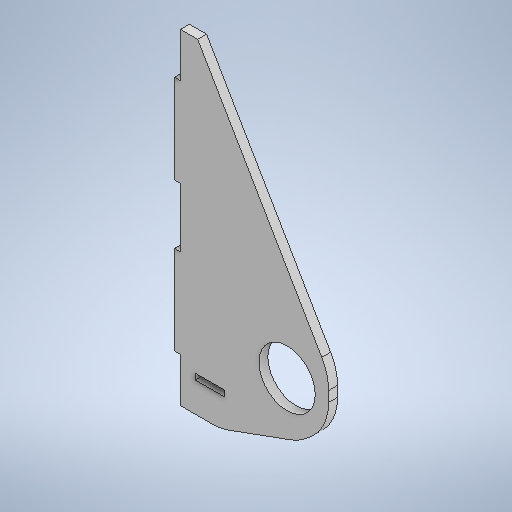
# Autodesk Inventor part: Piston_FloorHinge01
Saved by Autodesk Inventor 2025.2 (Build 292293000, 293)
## iProperties
Created: 2025-04-08
Part Number: Piston_FloorHinge01
Material: Generic
Document SubType Name: Sheet Metal
Designer: Victor
Density: 1 g/cm^3
Sheet Metal Rule: Default_mm
Appearance: Default
Author: Victor
Autodesk Inventor part; units mm, degrees
ref_plane "YZ Plane" through (0, 0, 0) normal (1, 0, 0) x (0, 1, 0)
ref_plane "XZ Plane" through (0, 0, 0) normal (0, 1, 0) x (-1, 0, 0)
ref_plane "XY Plane" through (0, 0, 0) normal (0, 0, 1) x (1, 0, 0)
sketch "Sketch1" plane through (0, 0, 0) normal (0, 0, 1) x (1, 0, 0)
  line L0 (-16.7671, 64.9713) -> (-16.7671, -55.0287)
  line L1 (-16.7671, -55.0287) -> (11.7813, -55.0287)
  line L2 (11.7813, -55.0287) -> (33.2329, -37.0287)
  line L3 (33.2329, -37.0287) -> (33.2329, -21.0287)
  line L4 (33.2329, -21.0287) -> (-16.7671, 64.9713)
  line L5 (-1.7671, -43.0287) -> (-11.7671, -43.0287)
  line L6 (-11.7671, -43.0287) -> (-11.7671, -45.0287)
  line L7 (-11.7671, -45.0287) -> (-1.7671, -45.0287)
  line L8 (-1.7671, -45.0287) -> (-1.7671, -43.0287)
  line L9 (-16.7671, -40.0287) -> (-18.7671, -40.0287)
  line L10 (-18.7671, -40.0287) -> (-18.7671, -10.0287)
  line L11 (-18.7671, -10.0287) -> (-16.7671, -10.0287)
  line L12 (-16.7671, -10.0287) -> (-16.7671, -40.0287)
  line L13 (-16.7671, 9.9713) -> (-18.7671, 9.9713)
  line L14 (-18.7671, 9.9713) -> (-18.7671, 39.9713)
  line L15 (-18.7671, 39.9713) -> (-16.7671, 39.9713)
  line L16 (-16.7671, 39.9713) -> (-16.7671, 9.9713)
  line L17 (-16.7671, 54.9713) -> (-10.9532, 54.9713)
  circle A0 centre (19.2329, -29.0287) radius 9.5
  line L18 (19.2329, -29.0287) -> (33.2329, -29.0287)
  point P0 (0, 0)
  point P1 (-17.7671, -40.0287)
  point P2 (-17.7671, -10.0287)
  dimension "d0" = 120
  dimension "d1" = 10
  dimension "d2" = 2
  dimension "d3" = 10
  dimension "d4" = 5
  dimension "d5" = 2
  dimension "d6" = 30
  dimension "d7" = 15
  dimension "d8" = 2
  dimension "d9" = 30
  dimension "d10" = 20
  dimension "d11" = 18
  dimension "d12" = 16
  dimension "d13" = 50
  dimension "d14" = 10
  dimension "d15" = 50
  dimension "d16" = 19
  dimension "d17" = 36
  dimension "d18" = 90
  measures "d0" distance of L0.start L0.end
  measures "d1" distance of L7.end L7.start
  measures "d2" distance of L7.start L5.end
  measures "d3" distance between parallel lines of L1 L7
  measures "d4" distance between parallel lines of L0 L6
  measures "d5" distance of L11.start L11.end
  measures "d6" distance of L10.start L11.start
  measures "d7" distance from line of L1 point (-17.767, -40.029)
  measures "d8" distance of L14.end L16.start
  measures "d9" distance of L14.start L14.end
  measures "d10" distance from line of point (-17.767, -10.029) L13
  measures "d11" distance from line of L2.end L1
  measures "d12" distance of L2.end L4.start
  measures "d13" distance between parallel lines of L12 L3
  measures "d14" distance from line of L0.start L17
  measures "d15" angle of L0 L2
  measures "d16" diameter of A0
  measures "d17" distance from line of L12 L18.start
  measures "d18" angle of L3 L18
extrude "Plate1" add sketch "Sketch1" along normal blind 3 contours L17 L4 L3 L2 L1 L0 | L0 L13 L14 L15 | L0 L9 L10 L11
chamfer "Corner Chamfer1" distance 15 angle 45 1 edges at (11.7813, -55.0287, 1.5)
fillet "Corner Round1" radius 17 4 edges at (33.2329, -37.0287, 1.5) (33.2329, -21.0287, 1.5) (23.272, -45.3869, 1.5) (-3.2187, -55.0287, 1.5)
equation "\"d2\" = d19"
equation "\"d5\" = d19"
equation "\"d8\" = d19"
equation "\"d21\" = Thickness"
equation "\"Thickness\" = plate_thickness"
equation "\"BendRadius\" = Thickness"
equation "\"BendReliefWidth\" = Thickness"
equation "\"BendReliefDepth\" = 0.5 * Thickness"
equation "\"CornerReliefSize\" = 4 * Thickness"
equation "\"MinimumRemnant\" = 2 * Thickness"
equation "\"TransitionRadius\" = BendRadius"
equation "\"JacobiRadiusSize\" = BendRadius"
equation "\"GapSize\" = Thickness"
equation "\"A_width\" = 46"
equation "\"A_joint_diameter\" = 16"
equation "\"A_joint_tolerance\" = 3"
equation "\"l___________\" = 0"
equation "\"l__________\" = 0"
equation "\"l_________\" = 0"
equation "\"rivet_diameter\" = 3.35"
equation "\"plate_thickness\" = 3"
equation "\"l________\" = 0"
equation "\"L_Piston_Top\" = 25"
equation "\"L_Piston_Bottom\" = 21"
equation "\"A_B_spacing\" = 2"
equation "\"thin_plate\" = 1.5"
equation "\"d19\" = 2"
body "Solid1"
